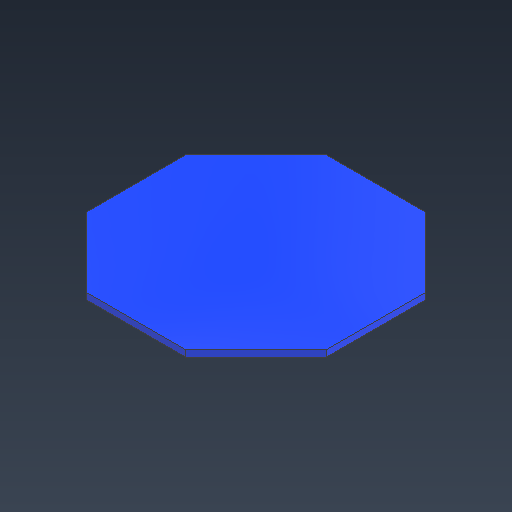
# Autodesk Inventor part: GPS-Compass_plexi
Saved by Autodesk Inventor 2026.2 (Build 302298000, 298)
## iProperties
Created: 2025-11-19
Part Number: GPS-Compass_plexi
Material: Generic
Document SubType Name: Modeling
Designer: MenMe
Density: 1 g/cm^3
Appearance: Default
Author: MenMe
Autodesk Inventor part; units mm, degrees
ref_plane "YZ Plane" through (0, 0, 0) normal (1, 0, 0) x (0, 1, 0)
ref_plane "XZ Plane" through (0, 0, 0) normal (0, 1, 0) x (-1, 0, 0)
ref_plane "XY Plane" through (0, 0, 0) normal (0, 0, 1) x (1, 0, 0)
sketch "Sketch1" plane through (0, 0, 0) normal (0, 1, 0) x (-1, 0, 0)
  line L0 (15.3073, 36.9552) -> (36.9552, 15.3073)
  line L1 (36.9552, 15.3073) -> (36.9552, -15.3073)
  line L2 (36.9552, -15.3073) -> (15.3073, -36.9552)
  line L3 (15.3073, -36.9552) -> (-15.3073, -36.9552)
  line L4 (-15.3073, -36.9552) -> (-36.9552, -15.3073)
  line L5 (-36.9552, -15.3073) -> (-36.9552, 15.3073)
  line L6 (-36.9552, 15.3073) -> (-15.3073, 36.9552)
  line L7 (-15.3073, 36.9552) -> (15.3073, 36.9552)
  point P0 (0, 0)
  point P1 (0, 0)
  point P2 (0, 0)
  dimension "d0" = 30.6147
  constraints: 16 end point, 2 coincident, 1 horizontal, 17 other
  measures "d0" distance of L6.end L0.start
extrude "Extrusion1" add sketch "Sketch1" along normal blind 2
body "Solid1"
